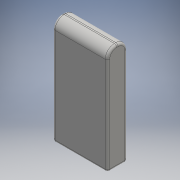
# Autodesk Inventor part: LIPO 1050
Saved by Autodesk Inventor 2016 (Build 200138000, 138)
## iProperties
Created: 2017-02-20
Part Number: LIPO 1050
Material: Generic
Document SubType Name: Modeling
Designer: jorge
Density: 1 g/cm^3
Appearance: Default
Author: jorge
Autodesk Inventor part; units mm, degrees
ref_plane "YZ Plane" through (0, 0, 0) normal (1, 0, 0) x (0, 1, 0)
ref_plane "XZ Plane" through (0, 0, 0) normal (0, 1, 0) x (-1, 0, 0)
ref_plane "XY Plane" through (0, 0, 0) normal (0, 0, 1) x (1, 0, 0)
sketch "Sketch1" plane through (0, 0, 0) normal (0, 1, 0) x (-1, 0, 0)
  line L0 (0, 0) -> (36, 0)
  line L1 (36, 0) -> (36, -70)
  line L2 (36, -70) -> (0, -70)
  line L3 (0, -70) -> (0, 0)
  dimension "d0" = 36
  dimension "d1" = 70
  constraints: 8 end point, 2 parallel, 1 horizontal, 1 perpendicular
  measures "d0" distance of L1.end L2.end
  measures "d1" distance of L0.end L1.end
extrude "Extrusion1" add sketch "Sketch1" along normal blind 13
fillet "Fillet1" radius 6 2 edges at (-18, 13, 0) (-18, 0, 0)
fillet "Fillet2" radius 1.5 14 edges at (0, 11.2426, -1.7574) (0, 6.5, 0) (0, 1.7574, -1.7574) (0, 0, -38) (0, 13, -38) (-36, 11.2426, -1.7574) (-36, 6.5, 0) (-36, 1.7574, -1.7574) (-36, 0, -38) (-36, 13, -38) (0, 6.5, -70) (-18, 13, -70) (-36, 6.5, -70) (-18, 0, -70)
body "Solid1"
